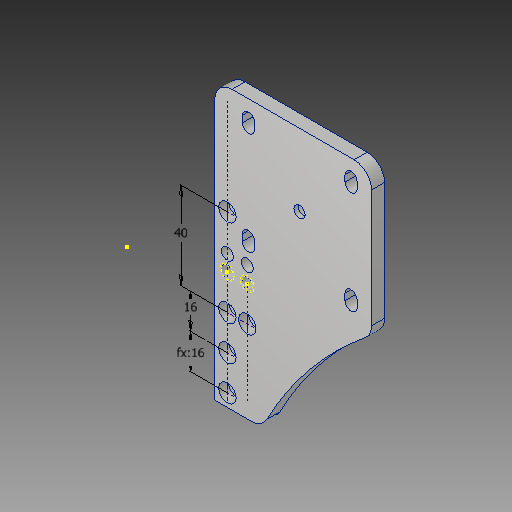
# Autodesk Inventor part: XMotorMount
Saved by Autodesk Inventor 2019 (Build 230136000, 136)
## iProperties
Created: 2018-10-14
Part Number: XMotorMount
Material: Aluminum 6061
Document SubType Name: Modeling
Designer: LillaHunden
Density: 2.7 g/cm^3
Appearance: Aluminum - Flat
Mass: 110.636 g
Surface Area: 179.852 cm^2
Volume: 40.9762 cm^3
Author: LillaHunden
Autodesk Inventor part; units mm, degrees
ref_plane "YZ Plane" through (0, 0, 0) normal (1, 0, 0) x (0, 1, 0)
ref_plane "XZ Plane" through (0, 0, 0) normal (0, 1, 0) x (-1, 0, 0)
ref_plane "XY Plane" through (0, 0, 0) normal (0, 0, 1) x (1, 0, 0)
sketch "Sketch1" plane through (0, 0, 0) normal (0, 0, 1) x (1, 0, 0)
  line L0 (112.0815, -40.6698) -> (40.0716, -40.6698)
  line L1 (40.0716, -40.6698) -> (40.0716, 86.9433)
  line L2 (40.0716, 86.9433) -> (112.0815, 86.9433)
  line L3 (112.0815, 86.9433) -> (112.0815, -40.6698)
  line L4 (40.0716, -40.6698) -> (50.0716, -40.6698) construction
  point P0 (0, 0)
  constraints: 8 end point, 2 parallel, 1 horizontal, 1 perpendicular
extrude "Extrusion1" add sketch "Sketch1" along normal blind 6
sketch "Sketch2" plane through (0, 0, 6) normal (0, 0, 1) x (1, 0, 0)
  point P0 (0, 0)
sketch "Sketch3" plane through (0, 0, 6) normal (0, 0, 1) x (1, 0, 0)
  circle A0 centre (45.9019, 20.4802) radius 3.25 construction
  circle A1 centre (55.0716, 20.4786) radius 3.25 construction
  circle A2 centre (55.0716, 13.1818) radius 3.25 construction
  circle A3 centre (45.9019, 13.1802) radius 3.25 construction
  line L0 (-8.5113, 9.3302) -> (60.0076, 9.3302) construction
  line L1 (60.0076, 9.3302) -> (60.0076, 24.3302) construction
  line L2 (-8.5113, 24.3302) -> (60.0076, 24.3302) construction
  line L3 (40.0716, 86.9433) -> (40.0716, -40.6698) projected
  line L4 (40.0716, 25.8302) -> (61.5076, 25.8302)
  line L5 (61.5076, 25.8302) -> (61.5076, 7.8302)
  line L6 (61.5076, 7.8302) -> (40.0716, 7.8302)
  line L7 (40.0716, 7.8302) -> (40.0716, 25.8302)
  line L8 (-8.5113, 9.3302) -> (-8.5113, 24.3302) projected
  point P0 (0, 0)
  point P1 (40.0716, -42.6698)
  dimension "d2" = 1.5
  dimension "d3" = 1.5
  dimension "d4" = 1.5
  constraints: 8 end point, 2 parallel, 1 horizontal, 1 perpendicular, 1 point on line
  measures "d2" distance between parallel lines of L0 L6
  measures "d3" distance between parallel lines of L4 L2
  measures "d4" distance between parallel lines of L5 L1
extrude "Extrusion2" [suppressed]
sketch "Sketch4" plane through (0, 0, 6) normal (0, 0, 1) x (1, 0, 0)
  circle A0 centre (102.6515, 97.6673) radius 2.8 construction
  circle A1 centre (55.5716, 78.9433) radius 2.8 construction
  circle A2 centre (55.5115, 50.5273) radius 2.8 construction
  circle A3 centre (102.6515, 50.5273) radius 2.8 construction
  line L0 (55.5716, 78.9433) -> (55.5716, 75.9433) construction
  line L1 (52.7716, 78.9433) -> (52.7716, 75.9433)
  line L2 (58.3716, 75.9433) -> (58.3716, 78.9433)
  arc A4 (58.3716, 78.9433) -> (52.7716, 78.9433) centre (55.5716, 78.9433) ccw
  arc A5 (52.7716, 75.9433) -> (58.3716, 75.9433) centre (55.5716, 75.9433) ccw
  line L3 (40.0716, 86.9433) -> (40.0716, -40.6698) projected
  line L4 (112.0815, 86.9433) -> (40.0716, 86.9433) projected
  point P0 (0, 0)
  point P1 (55.5716, 77.4433)
  point P2 (40.0716, -42.6698)
  dimension "d7" = 3
  dimension "d27" = 5.6
  dimension "d28" = 12.7
  dimension "d29" = 8
  constraints: 8 end point, 6 centre point, 4 point on circle, 4 tangent, 1 midpoint, 1 parallel, 1 vertical
  measures "d7" distance of L0.start L0.end
  measures "d27" distance between parallel lines of L1 L2
  measures "d28" distance between parallel lines of L3 L1
  measures "d29" distance from line of L4 L0.start
extrude "Extrusion3" cut sketch "Sketch4" against normal through all
pattern_linear "Rectangular Pattern1" count 2 spacing 47.14 along (1, 0, 0) count 2 spacing 47.14 along (0, -1, 0) of "Extrusion3"
sketch "Sketch7" plane through (0, 0, 6) normal (0, 0, 1) x (1, 0, 0)
  circle A0 centre (45.9019, 20.4802) radius 2.75
  circle A1 centre (55.0716, 13.1818) radius 2.45
  circle A2 centre (45.9019, 13.1802) radius 2.75
  circle A3 centre (55.0716, 20.4786) radius 2.75
  circle A4 centre (45.9019, 13.1802) radius 3.25 construction
  circle A5 centre (45.9019, 20.4802) radius 3.25 construction
  circle A6 centre (55.0716, 20.4786) radius 3.25 construction
  circle A7 centre (55.0716, 13.1818) radius 2.75 construction
  point P0 (0, 0)
  constraints: 4 centre point, 4 coincident
extrude "Extrusion6" cut sketch "Sketch7" against normal through all
sketch "Sketch8" plane through (0, 0, 6) normal (0, 0, 1) x (1, 0, 0)
  circle A0 centre (55.0716, 13.1818) radius 3.25 construction
  circle A1 centre (45.9019, 13.1802) radius 3.25 construction
  circle A2 centre (45.9019, 13.1802) radius 2.75 construction
  line L0 (45.9019, 13.1802) -> (45.9019, -34.9017) construction
  circle A3 centre (55.0716, 13.1818) radius 2.45 construction
  line L1 (55.0716, 13.1818) -> (55.0716, -34.9017) construction
  line L2 (45.9019, 13.1802) -> (45.9019, 82.3427) construction
  point P0 (0, 0)
  point P1 (45.9019, -2.9017)
  point P2 (45.9019, -18.9017)
  point P3 (55.0716, -2.9017)
  point P4 (45.9019, 37.0983)
  dimension "d30" = 16
  dimension "d31" = 16
  dimension "d32" = 40
  constraints: 6 end point, 4 point on line, 3 vertical, 1 coincident, 1 horizontal alignment
  measures "d30" distance of point (45.902, -2.902) point (45.902, -18.902)
  measures "d31" distance of point (45.902, -18.902) point (45.902, -34.902)
  measures "d32" distance of point (45.902, -2.902) point (45.902, 37.098)
sketch "Sketch9" plane through (0, 0, 6) normal (0, 0, 1) x (1, 0, 0)
  point P0 (55.0716, -2.9017)
  point P1 (45.9019, -2.9017)
  point P2 (45.9019, -18.9017)
  point P3 (45.9019, -34.9017)
  point P4 (45.9019, 37.0983)
hole "Hole1" at (55.0716, -2.9017, 6) at (45.9019, -2.9017, 6) at (45.9019, -18.9017, 6) at (45.9019, -34.9017, 6) at (45.9019, 37.0983, 6) direction (0, 0, -1) diameter 4.5 depth 6 counterbore diameter 8 counterbore depth 4.5
sketch "Sketch10" plane through (0, 0, 0) normal (0, 0, -1) x (-1, 0, 0)
  circle A0 centre (-79.0293, 53.7433) radius 5.55
  circle A1 centre (-79.0293, 53.7433) radius 2.5 projected
  point P0 (0, 0)
  dimension "d42" = 11.1
  constraints: 1 centre point
  measures "d42" diameter of A0
extrude "Extrusion7" cut sketch "Sketch10" against normal blind 4 contours A0 | A1
sketch "Sketch11" plane through (0, 0, 6) normal (0, 0, 1) x (1, 0, 0)
  circle A0 centre (79.0293, 53.7433) radius 2.5 construction
  circle A1 centre (79.0293, 53.7433) radius 2.6
  point P0 (0, 0)
  dimension "d47" = 5.2
  constraints: 1 centre point, 1 coincident
  measures "d47" diameter of A1
extrude "Extrusion8" cut sketch "Sketch11" against normal through all
sketch "Sketch12" plane through (0, 0, 6) normal (0, 0, 1) x (1, 0, 0)
  line L0 (40.0716, -40.6698) -> (112.0815, -40.6698) projected
  arc A0 (112.0815, 21.0326) -> (61.7828, -40.6698) centre (221.9091, -119.8494) ccw
  line L1 (112.0815, -40.6698) -> (112.0815, 86.9433) projected
  point P0 (0, 0)
  constraints: 2 point on circle, 2 point on line, 1 centre point
extrude "Extrusion9" cut sketch "Sketch12" against normal through all
fillet "Fillet1" radius 8 2 edges at (61.7828, -40.6698, 3) (112.0815, 21.0326, 3)
fillet "Fillet2" radius 8 2 edges at (112.0815, 86.9433, 3) (40.0716, 86.9433, 3)
equation "\"d31\" = d30"
body "Solid1"
